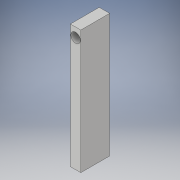
# Autodesk Inventor part: blde
Saved by Autodesk Inventor 2019 (Build 230136000, 136)
## iProperties
Created: 2020-02-26
Part Number: blde
Material: Generic
Document SubType Name: Sheet Metal
Designer: unusualgamer
Density: 1 g/cm^3
Sheet Metal Rule: Default_mm
Appearance: Default
Author: unusualgamer
Autodesk Inventor part; units mm, degrees
ref_plane "YZ Plane" through (0, 0, 0) normal (1, 0, 0) x (0, 1, 0)
ref_plane "XZ Plane" through (0, 0, 0) normal (0, 1, 0) x (-1, 0, 0)
ref_plane "XY Plane" through (0, 0, 0) normal (0, 0, 1) x (1, 0, 0)
sketch "Sketch1" plane through (0, 0, 0) normal (1, 0, 0) x (0, 1, 0)
  line L0 (12.1919, 24.5577) -> (-64.8081, 24.5577)
  line L1 (-64.8081, 24.5577) -> (-64.8081, 6.5577)
  line L2 (-64.8081, 6.5577) -> (12.1919, 6.5577)
  line L3 (12.1919, 6.5577) -> (12.1919, 24.5577)
  point P0 (0, 0)
  dimension "d0" = 77
  dimension "d1" = 18
  measures "d0" distance of L2.end L1.end
  measures "d1" distance of L1.end L0.end
extrude "Plate1" add sketch "Sketch1" along normal blind 6.5
sketch "Sketch2" plane through (0, -64.8081, 24.5577) normal (0, 0, 1) x (1, 0, 0)
  point P0 (0, 64.8081)
  point P1 (3.3009, 71.2411)
hole "Hole1" at (3.3009, 6.4331, 24.5577) direction (0, 0, -1) diameter 6 end through all
equation "\"d8\" = Thickness"
equation "\"d2\" = Thickness"
equation "\"BendRadius\" = Thickness"
equation "\"BendReliefWidth\" = Thickness"
equation "\"BendReliefDepth\" = 0.5 * Thickness"
equation "\"CornerReliefSize\" = 4 * Thickness"
equation "\"MinimumRemnant\" = 2 * Thickness"
equation "\"TransitionRadius\" = BendRadius"
equation "\"JacobiRadiusSize\" = BendRadius"
equation "\"GapSize\" = Thickness"
equation "\"Thickness\" = 6.5"
body "Solid1"
